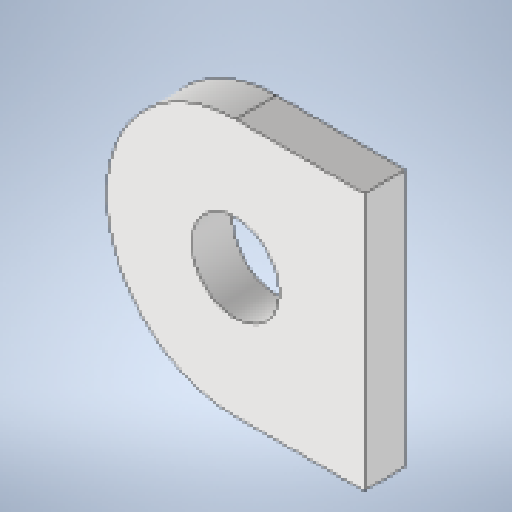
# Autodesk Inventor part: PNS-0872 roof ring
Saved by Autodesk Inventor 2025.1 (Build 291241020, 241B)
## iProperties
Created: 2024-05-23
Part Number: PNS-0872 roof ring
Material: Generic
Document SubType Name: Sheet Metal
Designer: user
Mass: 0.559799 g
Surface Area: 23.3947 cm^2
Volume: 0.559799 cm^3
Density: 1 g/cm^3
Flat Pattern Width: 5 cm
Flat Pattern Length: 5 cm
Flat Pattern Area: 25 cm^2
Sheet Metal Rule: Default_mm
Sheet Metal Width: 50.000 mm
Sheet Metal Length: 50.000 mm
Sheet Metal Area: 2500.000 mm^2
Appearance: Default
Author: admin
Autodesk Inventor part; units mm, degrees
ref_plane "YZ Plane" through (0, 0, 0) normal (1, 0, 0) x (0, 1, 0)
ref_plane "XZ Plane" through (0, 0, 0) normal (0, 1, 0) x (-1, 0, 0)
ref_plane "XY Plane" through (0, 0, 0) normal (0, 0, 1) x (1, 0, 0)
sketch "Sketch1" plane through (0, 0, 0) normal (0, 0, 1) x (1, 0, 0)
  line L0 (-25, 25) -> (25, 25)
  line L1 (25, 25) -> (25, -25)
  line L2 (25, -25) -> (-25, -25)
  line L3 (-25, -25) -> (-25, 25)
  line L4 (-25, 25) -> (25, -25) construction
  line L5 (25, 25) -> (-25, -25) construction
  circle A0 centre (0, 0) radius 8.5
  line L6 (0, 25) -> (0, -25) construction
  arc A1 (0, 25) -> (0, -25) centre (0, 0) ccw
  point P0 (0, 0)
  point P1 (-25, 0)
  dimension "d0" = 50
  dimension "d1" = 50
  dimension "d14" = 17
  measures "d0" distance of L1.end L2.end
  measures "d1" distance of L0.end L1.end
  measures "d14" diameter of A0
extrude "Plate1" add sketch "Sketch1" along normal blind 8 contours L0 L1 L2 A1
equation "\"d2\" = Thickness"
equation "\"BendRadius\" = Thickness"
equation "\"BendReliefWidth\" = Thickness"
equation "\"BendReliefDepth\" = 0.5 * Thickness"
equation "\"CornerReliefSize\" = 4 * Thickness"
equation "\"MinimumRemnant\" = 2 * Thickness"
equation "\"TransitionRadius\" = BendRadius"
equation "\"JacobiRadiusSize\" = BendRadius"
equation "\"GapSize\" = Thickness"
equation "\"Thickness\" = 8"
body "Solid1"
